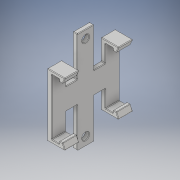
# Autodesk Inventor part: Eraser Holder
Saved by Autodesk Inventor 2019 (Build 230136000, 136)
## iProperties
Created: 2019-06-11
Part Number: Eraser Holder
Material: Generic
Document SubType Name: Modeling
Designer: Matthew XPS
Density: 1 g/cm^3
Appearance: Default
Author: Matthew XPS
Autodesk Inventor part; units mm, degrees
sketch "Sketch1" plane through (0, 0, 0) normal (1, 0, 0) x (0, 1, 0)
  line L0 (0, 0) -> (51.2, 0)
  line L1 (51.2, 0) -> (51.2, -13)
  line L2 (51.2, -13) -> (0, -13)
  line L3 (0, -13) -> (0, 0)
  dimension "d0" = 51.2
  dimension "d1" = 13
  constraints: 8 end point, 2 parallel, 1 horizontal, 1 perpendicular
  measures "d0" distance of L1.end L2.end
  measures "d1" distance of L0.end L1.end
extrude "Extrusion1" add sketch "Sketch1" along normal blind 4
sketch "Sketch3" plane through (4, 0, 0) normal (1, 0, 0) x (0, 0, -1)
  line L0 (0, 51.2) -> (0, 0) projected
  line L1 (0, 51.2) -> (13, 51.2)
  line L2 (13, 51.2) -> (13, 54.2)
  line L3 (13, 54.2) -> (0, 54.2)
  line L4 (0, 54.2) -> (0, 51.2)
  dimension "d4" = 13
  dimension "d5" = 3
  constraints: 8 end point, 2 parallel, 1 horizontal, 1 perpendicular
  measures "d4" distance of L3.end L2.end
  measures "d5" distance of L2.end L1.end
extrude "Extrusion2" add sketch "Sketch3" along normal blind 6.9
sketch "Sketch4" plane through (4, 0, 0) normal (-1, 0, 0) x (0, 0, 1)
  line L0 (-13, 51.2) -> (0, 51.2) projected
  line L1 (0, 54.2) -> (0, 51.2) projected
  line L2 (-13, 54.2) -> (0, 54.2) projected
  line L3 (-13, 51.2) -> (-13, 54.2) projected
  point P0 (0, 0)
extrude "Extrusion3" add sketch "Sketch4" along normal blind 4
sketch "Sketch5" plane through (0, 0, 0) normal (0, 0, 1) x (1, 0, 0)
  line L0 (10.9, 54.2) -> (10.9, 51.2) projected
  line L1 (10.9, 51.2) -> (10.9, 49)
  line L2 (10.9, 49) -> (13.9, 49)
  line L3 (13.9, 49) -> (16.2152, 54.2)
  line L4 (13.9, 49) -> (19.5921, 49) construction
  line L5 (16.2152, 54.2) -> (10.9, 54.2)
  point P0 (0, 0)
  dimension "d10" = 2.2
  dimension "d11" = 3
  dimension "d12" = 66
  constraints: 10 end point, 2 horizontal, 1 equal length, 1 perpendicular, 1 vertical
  measures "d10" distance of L0.end L1.end
  measures "d11" distance of L1.end L2.end
  measures "d12" angle of L4 L3
extrude "Extrusion4" add sketch "Sketch5" against normal up to surface (13 mm away)
ref_plane "Work Plane2" through (4, 25.6, -13) normal (0, -1, 0) x (1, 0, 0)
mirror "Mirror1" about plane through (4, 25.6, -13) normal (0, -1, 0) of "Extrusion2", "Extrusion3", "Extrusion4"
sketch "Sketch6" plane through (10.9, 49, 0) normal (0, 0, 1) x (1, 0, 0)
  line L0 (-6.9, 2.2) -> (-6.9, -49) projected
  line L1 (-6.9, -23.4) -> (-10.9, -23.4)
  line L2 (-10.9, -33.4) -> (-10.9, -13.4)
  line L3 (-10.9, -13.4) -> (-6.9, -13.4)
  line L4 (-6.9, -13.4) -> (-6.9, -33.4)
  line L5 (-6.9, -33.4) -> (-10.9, -33.4)
  line L6 (-10.9, -33.4) -> (-6.9, -13.4) construction
  line L7 (-10.9, -13.4) -> (-6.9, -33.4) construction
  point P0 (-10.9, -49)
  point P1 (-8.9, -23.4)
  dimension "d15" = 20
  constraints: 14 end point, 4 midpoint, 2 parallel, 2 perpendicular, 1 horizontal
  measures "d15" distance of L2.start L2.end
extrude "Extrusion5" add sketch "Sketch6" along normal blind 36
ref_plane "Work Plane3" through (10.9, 49, 18) normal (0, 0, 1) x (1, 0, 0)
mirror "Mirror2" about plane through (10.9, 49, 18) normal (0, 0, 1) of "Extrusion2", "Extrusion3", "Extrusion4", "Mirror1", "Extrusion1"
sketch "Sketch7" plane through (0, 15.6, 0) normal (0, -1, 0) x (1, 0, 0)
  line L0 (0, 0) -> (0, 36) projected
  line L1 (0, 18) -> (4, 18)
  line L2 (4, 0) -> (4, 36) projected
  line L3 (4, 10.5) -> (0, 10.5)
  line L4 (0, 10.5) -> (0, 25.5)
  line L5 (0, 25.5) -> (4, 25.5)
  line L6 (4, 25.5) -> (4, 10.5)
  line L7 (4, 10.5) -> (0, 25.5) construction
  line L8 (0, 10.5) -> (4, 25.5) construction
  point P0 (2, 18)
  dimension "d18" = 4
  dimension "d19" = 15
  constraints: 14 end point, 5 midpoint, 2 parallel, 1 horizontal, 1 perpendicular
  measures "d18" distance of L4.end L5.end
  measures "d19" distance of L3.end L4.end
extrude "Extrusion6" add sketch "Sketch7" along normal blind 36
sketch "Sketch8" plane through (0, 0, 0) normal (-1, 0, 0) x (0, 0, 1)
  line L0 (25.5, -20.4) -> (10.5, -20.4) projected
  line L1 (10.5, -20.4) -> (10.5, -5.4)
  line L2 (10.5, -5.4) -> (25.5, -5.4)
  line L3 (25.5, -5.4) -> (25.5, -20.4)
  circle A0 centre (18, -12.9) radius 3.15
  point P0 (0, 0)
  dimension "d22" = 6.3
  constraints: 6 end point, 3 perpendicular, 1 centre point, 1 horizontal
  measures "d22" diameter of A0
extrude "Extrusion7" cut sketch "Sketch8" against normal blind 36 contours A0
ref_plane "Work Plane4" through (0, 25.6, 0) normal (0, 1, 0) x (1, 0, 0)
mirror "Mirror3" about plane through (0, 25.6, 0) normal (0, 1, 0) of "Extrusion7", "Extrusion6"
fillet "Fillet1" radius 0.5 110 edges at (2, 35.6, 10.5) (2, 71.6, 10.5) (4, 64.1, 14.85) (0, 64.1, 14.85) (2, 35.6, 25.5) (0, 53.6, 10.5) (4, 71.6, 18) (0, 71.6, 18) (2, 71.6, 25.5) (4, 53.6, 25.5) (0, 53.6, 25.5) (4, 53.6, 10.5) (4, 7.8, 0) (2, 15.6, 0) (0, 6.3, 0) (4, 15.6, 5.25) (0, 15.6, 5.25) (2, 15.6, 10.5) (0, -12.9, 14.85) (4, -12.9, 14.85) (4, -2.4, 10.5) (0, -2.4, 10.5) (0, -20.4, 18) (2, -20.4, 25.5) (4, -2.4, 25.5) (0, -2.4, 25.5) (2, 15.6, 25.5) (4, 7.8, 36) (4, 43.4, 36) (2, 15.6, 36) (0, 6.3, 36) (12.4, 2.2, 36) (15.0576, -0.4, 36) (13.9, 2.2, 42.5) (12.4, 2.2, 49) (15.0576, -0.4, 49) (0, -3, 42.5) (8.1076, -3, 49) (8.1076, -3, 36) (7.45, 0, 49) (7.45, 0, 36) (4, 0, 42.5) (10.9, 0, 42.5) (10.9, 1.1, 36) (10.9, 2.2, 42.5) (10.9, 1.1, 49) (16.2152, -3, 42.5) (7.45, 0, -13) (4, 0, -6.5) (8.1076, -3, -13) (0, -3, -6.5) (16.2152, -3, -6.5) (15.0576, -0.4, -13) (7.45, 0, 0) (10.9, 1.1, 0) (12.4, 2.2, 0) (15.0576, -0.4, 0) (8.1076, -3, 0) (10.9, 2.2, -6.5) (10.9, 0, -6.5) (10.9, 1.1, -13) (12.4, 2.2, -13) (13.9, 2.2, -6.5) (7.45, 51.2, -13) (4, 51.2, -6.5) (0, 54.2, -6.5) (8.1076, 54.2, -13) (16.2152, 54.2, -6.5) (15.0576, 51.6, -13) (13.9, 49, -6.5) (0, 35.6, 5.25) (4, 35.6, 5.25) (0, 44.9, 0) (4, 43.4, 0) (2, 35.6, 0) (10.9, 50.1, 0) (7.45, 51.2, 0) (12.4, 49, 0) (8.1076, 54.2, 0) (15.0576, 51.6, 0) (10.9, 49, -6.5) (10.9, 51.2, -6.5) (10.9, 50.1, -13) (12.4, 49, -13) (4, 25.6, -13) (0, 25.6, -13) (0, 15.6, 30.75) (4, 15.6, 30.75) (2, 35.6, 36) (4, 35.6, 30.75) (0, 35.6, 30.75) (12.4, 49, 36) (13.9, 49, 42.5) (10.9, 49, 42.5) (12.4, 49, 49) (7.45, 51.2, 36) (10.9, 50.1, 36) (10.9, 50.1, 49) (10.9, 51.2, 42.5) (4, 25.6, 49) (7.45, 51.2, 49) (4, 51.2, 42.5) (0, 44.9, 36) (8.1076, 54.2, 36) (15.0576, 51.6, 36) (0, 25.6, 49) (8.1076, 54.2, 49) (0, 54.2, 42.5) (16.2152, 54.2, 42.5) (15.0576, 51.6, 49)
body "Solid1"
